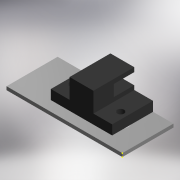
# Autodesk Inventor part: Z-linear-encoder
Saved by Autodesk Inventor 2016 (Build 200138000, 138)
## iProperties
Created: 2015-05-21
Part Number: Z-linear-encoder
Material: Generic
Document SubType Name: Modeling
Designer: as
Mass: 0.931304 g
Surface Area: 8.80296 cm^2
Volume: 0.931304 cm^3
Density: 1 g/cm^3
Appearance: Default
Author: as
Autodesk Inventor part; units mm, degrees
ref_plane "YZ Plane" through (0, 0, 0) normal (1, 0, 0) x (0, 1, 0)
ref_plane "XZ Plane" through (0, 0, 0) normal (0, 1, 0) x (-1, 0, 0)
ref_plane "XY Plane" through (0, 0, 0) normal (0, 0, 1) x (1, 0, 0)
sketch "Sketch1" plane through (0, 0, 0) normal (0, 0, 1) x (1, 0, 0)
  point P0 (0, 0)
sketch "Sketch2" plane through (0, 0, 0) normal (0, 0, 1) x (1, 0, 0)
  line L0 (0, 0) -> (-34, 0)
  line L1 (-34, 0) -> (-34, 15)
  line L2 (-34, 15) -> (0, 15)
  line L3 (0, 15) -> (0, 0)
  dimension "d0" = 34
  dimension "d1" = 15
  constraints: 8 end point, 2 parallel, 1 horizontal, 1 perpendicular
  measures "d0" distance of L1.end L2.end
  measures "d1" distance of L0.end L1.end
extrude "Extrusion1" add sketch "Sketch2" along normal blind 1
sketch "Sketch3" plane through (0, 0, 1) normal (0, 0, 1) x (1, 0, 0)
  line L0 (0, 0) -> (0, 15) projected
  point P0 (-8, 7.5)
  point P1 (-22, 7.5)
  dimension "d4" = 14
  dimension "d5" = 8
  measures "d4" distance of point (-8, 7.5) point (-22, 7.5)
  measures "d5" distance from line of L0 point (-8, 7.5)
hole "Hole1" at (-22, 7.5, 1) at (-8, 7.5, 1) direction (0, 0, -1) diameter 4.5 end through all
sketch "Sketch4" plane through (0, 0, 1) normal (0, 0, 1) x (1, 0, 0)
  line L0 (-24, 15) -> (-6, 15)
  line L1 (-6, 15) -> (-6, 3)
  line L2 (-6, 3) -> (-24, 3)
  line L3 (-24, 3) -> (-24, 15)
  line L4 (0, 0) -> (0, 15) projected
  dimension "d13" = 18
  dimension "d14" = 12
  dimension "d15" = 6
  constraints: 8 end point, 2 parallel, 1 horizontal, 1 perpendicular
  measures "d13" distance of L1.end L2.end
  measures "d14" distance of L0.end L1.end
  measures "d15" distance between parallel lines of L4 L1
extrude "Extrusion2" add sketch "Sketch4" along normal blind 2.8
sketch "Sketch6" plane through (0, 0, 3.8) normal (0, 0, 1) x (1, 0, 0)
  arc A0 (-24, 6.4692) -> (-24, 8.5308) centre (-22, 7.5) ccw projected
  arc A1 (-6, 8.5308) -> (-6, 6.4692) centre (-8, 7.5) ccw projected
  point P0 (0, 0)
  constraints: 2 coincident
hole "Hole2" at (-8, 7.5, 3.8) at (-22, 7.5, 3.8) direction (0, 0, -1) diameter 2 end through all
sketch "Sketch5" plane through (0, 0, 3.8) normal (0, 0, 1) x (1, 0, 0)
  line L0 (-34, 15) -> (0, 15) projected
  line L1 (-18.5, 15) -> (-11.5, 15)
  line L2 (-11.5, 15) -> (-11.5, 3)
  line L3 (-11.5, 3) -> (-18.5, 3)
  line L4 (-18.5, 3) -> (-18.5, 15)
  line L5 (-24, 15) -> (-24, 3) projected
  line L6 (-6, 3) -> (-6, 15) projected
  point P0 (0, 0)
  dimension "d18" = 7
  dimension "d19" = 0
  dimension "d20" = 5.5
  dimension "d21" = 5.5
  constraints: 8 end point, 2 parallel, 1 collinear, 1 perpendicular, 1 point on line
  measures "d18" distance of L1.start L1.end
  measures "d19" vertical distance of L1.start L1.end
  measures "d20" distance between parallel lines of L5 L4
  measures "d21" distance between parallel lines of L6 L2
extrude "Extrusion3" add sketch "Sketch5" along normal blind 5.8
sketch "Sketch7" plane through (-34, 15, 0) normal (0, 1, 0) x (1, 0, 0)
  line L0 (0, 0) -> (34, 0) projected
  line L1 (0, 0) -> (0, -1) projected
  line L2 (10, -1) -> (0, -1) projected
  line L3 (10, -1) -> (10, -3.8) projected
  line L4 (15.5, -3.8) -> (10, -3.8) projected
  line L5 (15.5, -3.8) -> (15.5, -9.6) projected
  line L6 (22.5, -9.6) -> (15.5, -9.6) projected
  line L7 (22.5, -3.8) -> (22.5, -9.6) projected
  line L8 (28, -3.8) -> (22.5, -3.8) projected
  line L9 (28, -1) -> (28, -3.8) projected
  line L10 (34, -1) -> (28, -1) projected
  line L11 (34, 0) -> (34, -1) projected
  line L12 (15.5, -3.8) -> (15.5, -9.6) projected
  line L13 (22.5, -8.35) -> (15.5, -8.35)
  line L14 (15.5, -8.35) -> (15.5, -5)
  line L15 (15.5, -5) -> (22.5, -5)
  line L16 (22.5, -5) -> (22.5, -8.35)
  dimension "d31" = 5
  dimension "d32" = 1.25
  constraints: 8 end point, 2 parallel, 2 point on line, 1 horizontal, 1 perpendicular
  measures "d31" distance between parallel lines of L0 L15
  measures "d32" distance between parallel lines of L6 L13
extrude "Extrusion4" cut sketch "Sketch7" against normal blind 6 contours L15 L7 L13 L5
sketch "Sketch8" plane through (0, 0, 1) normal (0, 0, 1) x (1, 0, 0)
  point P0 (0, 0)
fillet "Fillet1" radius 1 8 edges at (-34, 0, 0.5) (0, 0, 0.5) (0, 15, 0.5) (-34, 15, 0.5) (-6, 15, 2.4) (-6, 3, 2.4) (-24, 15, 2.4) (-24, 3, 2.4)
move faces "Move1" translate (0, 0, 1) faces at (-18.4872, 1.7718, 0)
body "Solid1"
